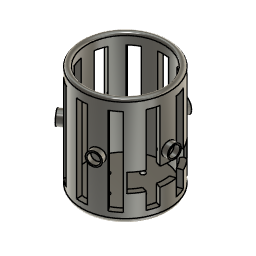
DRONE_V12 v0 (Autodesk Fusion 360 archive; units mm, degrees)
design "Final_motor"
Autodesk Fusion 360 part; units mm, degrees
sketch "Sketch1" plane through (0, 0, 0) normal (0, 0, 1) x (1, 0, 0)
  circle A0 centre (0, 0) radius 14
  circle A1 centre (0, 0) radius 16
  line L0 (0, 5.5) -> (0, 6.5)
  circle A2 centre (0, 6.5) radius 1
  circle A3 centre (-6.5, 0) radius 1
  circle A4 centre (0, -6.5) radius 1
  circle A5 centre (6.5, 0) radius 1
  dimension "d2" = 28
  dimension "d3" = 6.5
  dimension "d4" = 2
  dimension "d6" = 360
  constraint coincident A0.centre A1.centre
  constraint vertical L0
  constraint coincident L0.end A2.centre
  constraint coincident A2 L0.start
  measures "d2" diameter of A0
  measures "d3" distance of A0.centre L0.end
  measures "d4" diameter of A2
extrude "Extrude1" add sketch "Sketch1" along normal blind 2 contours A0
thread "Thread1" "ISO Metric profile 2.0 M2x0.25 6H" major diameter 2.0555 minor diameter 1.7694 pitch 0.25 angle 60 resizes the face on face at (7.4988, -0.0498, 1.3333)
thread "Thread2" "ISO Metric profile 2.0 M2x0.25 6H" major diameter 2.0555 minor diameter 1.7694 pitch 0.25 angle 60 resizes the face on face at (0.995, 6.4004, 0.6667)
thread "Thread3" "ISO Metric profile 2.0 M2x0.25 6H" major diameter 2.0555 minor diameter 1.7694 pitch 0.25 angle 60 resizes the face on face at (-5.5012, 0.0498, 0.6667)
thread "Thread4" "ISO Metric profile 2.0 M2x0.25 6H" major diameter 2.0555 minor diameter 1.7694 pitch 0.25 angle 60 resizes the face on face at (0.995, -6.4004, 1.3333)
sketch "Sketch2" plane through (0, 0, 2) normal (0, 0, 1) x (-1, 0, 0)
  circle A0 centre (-6.5, 0) radius 0.8847
  circle A1 centre (6.5, 0) radius 0.8847
  circle A2 centre (0, -6.5) radius 0.8847
  circle A3 centre (0, 6.5) radius 0.8847
  circle A4 centre (0, 0) radius 14
  circle A5 centre (0, 0) radius 16
  circle A6 centre (0, 0) radius 14
  constraint concentric A4 A5
  constraint concentric A5 A6
extrude "Extrude2" add sketch "Sketch2" along normal blind 38 and the other way blind 2 contours A5
sketch "Sketch3" plane through (0, 0, 0) normal (1, 0, 0) x (0, 1, 0)
  line L0 (11, 10) -> (-11, 10)
  line L1 (-11, 10) -> (-11, 16.725)
  line L2 (-11, 16.725) -> (11, 16.725)
  line L3 (11, 16.725) -> (11, 10)
  line L4 (11, 10) -> (-11, 16.725) construction
  line L5 (-11, 10) -> (11, 16.725) construction
  point P0 (0, 13.3625)
  constraint horizontal L0
  constraint perpendicular L0 L1
  constraint parallel L0 L2
  constraint parallel L1 L3
  constraint coincident L4 P0
  constraint coincident L5 P0
extrude "Extrude3" cut sketch "Sketch3" along normal through all
sketch "Sketch4" plane through (0, 0, 0) normal (0, 1, 0) x (1, 0, 0)
  line L0 (2, -36) -> (-2, -36)
  line L1 (-2, -36) -> (-2, -4)
  line L2 (-2, -4) -> (2, -4)
  line L3 (2, -4) -> (2, -36)
  constraint horizontal L0
  constraint vertical L1
  constraint horizontal L2
  constraint vertical L3
extrude "Extrude4" cut sketch "Sketch4" along normal blind 19
pattern_circular "C-Pattern1" count 10 over 360 about axis through (0, 0, 1.75) along (0, 0, 1) of "Extrude4"
fillet "Fillet1" radius 2 1 edges at (14.9172, -5.7858, 0)
fillet "Fillet2" radius 1 1 faces at (-15.2216, 1.4904, 40)
sketch "Sketch5" plane through (0, 0, 0) normal (1, 0, 0) x (0, 1, 0)
  circle A0 centre (0, 5) radius 2.5
  circle A1 centre (0, 5) radius 2
  dimension "d30" = 5
  dimension "d31" = 4
  constraint concentric A0 A1
  measures "d30" diameter of A0
  measures "d31" diameter of A1
extrude "Extrude5" add sketch "Sketch5" along normal blind 18 and the other way blind -14
move_face "MoveFace1" to x (1, 0, 0) y (0, 1, 0) z (0, 0, 1) at (0, 0, 16) 8 faces at (14.0782, -2.4989, 4.9257) (14, -2.462, 5.0578) (17.2681, 2.4935, 4.8201) (15.9996, 0.1099, 4.3399) (14, 2.462, 4.9422) (14.0871, 2.4995, 5.0493) (18, 2.3166, 4.7764) (17.2918, 1.994, 4.8446)
pattern_circular "C-Pattern2" count 5 over 360 about axis through (0, 0, 1.75) along (0, 0, 1) of 8 faces at (14, 2.462, 20.9422) (18, 2.3166, 20.7764) (17.2918, 1.994, 20.8446) (14.0782, -2.4989, 20.9257) (14.0871, 2.4995, 21.0493) (17.2681, 2.4935, 20.8201) (14, -2.462, 21.0578) (15.9996, 0.1064, 20.3395)
sketch "Sketch6" plane through (0, 0, 0) normal (0, 0, 1) x (1, 0, 0)
  circle A0 centre (0, 0) radius 133.35
  circle A1 centre (0, 0) radius 139.7
  dimension "d38" = 266.7
  dimension "d39" = 279.4
  constraint coincident A0.centre A1.centre
  constraint concentric A0 A1
  measures "d38" diameter of A0
  measures "d39" diameter of A1
extrude "Extrude6" [rolled back] along distance 40 taper angle 0
sketch "Sketch7" plane through (5.5623, -17.119, 0) normal (0.309017, -0.951057, 0) x (0.951057, 0.309017, 0)
  circle A0 centre (0, 21) radius 2
  circle A1 centre (0, 21) radius 2.5
  circle A2 centre (0, 21) radius 2
  constraint concentric A0 A2
extrude "Extrude1'" [rolled back] along distance 139.7 taper angle 0 in component "Component"
component_pattern "component pattern"
sketch "Sketch8" plane through (0, 0, 40) normal (0, 0, 1) x (-1, 0, 0)
  circle A0 centre (0, 0) radius 133.35
  circle A1 centre (0, 0) radius 139.7
  circle A2 centre (0, 0) radius 139.7
  circle A3 centre (0, 0) radius 184.8239
  constraint coincident A0.centre A1.centre
extrude "Extrude2'" [rolled back] along distance -180 taper angle 0 in component "Component"
